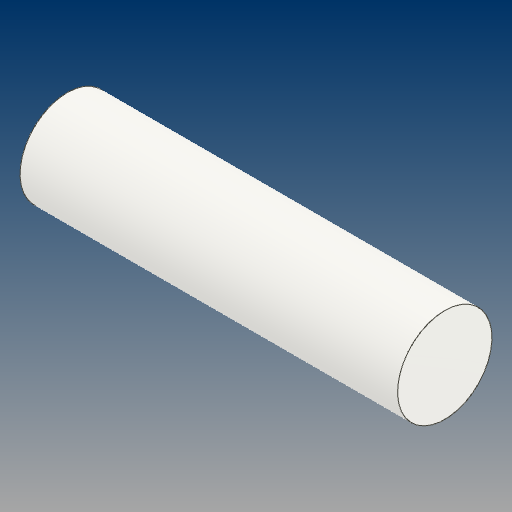
# Autodesk Inventor part: Shaft
Saved by Autodesk Inventor 2020 (Build 240168000, 168)
## iProperties
Created: 2020-09-14
Part Number: Shaft
Material: Steel
Document SubType Name: Modeling
Designer: alons
Density: 1 g/cm^3
Appearance: Steel
CustomPartVersion: 1
Author: alons
Length: 2.000 mm
Autodesk Inventor part; units mm, degrees
ref_plane "Start Plane" through (0, 0, 0) normal (1, 0, 0) x (0, 1, 0)
ref_plane "XZ Plane" through (0, 0, 0) normal (0, 1, 0) x (-1, 0, 0)
ref_plane "XY Plane" through (0, 0, 0) normal (0, 0, 1) x (1, 0, 0)
sketch "Main Sketch" plane through (0, 0, 0) normal (0, 0, 1) x (1, 0, 0)
  line L0 (0, 0) -> (2, 0)
  line L1 (0, 0) -> (0, 0.25)
  line L2 (2, 0.25) -> (2, 0)
  line L3 (0, 0.25) -> (2, 0.25)
  dimension "d3" = 0.5
  constraints: 8 end point, 3 horizontal, 2 vertical
  measures "d3" diameter of L3 L0
revolve "Revolution1" add sketch "Main Sketch" angle 360 about axis through (0, 0, 0) along (1, 0, 0)
equation "\"Length\" = 2"
body "Solid1"
